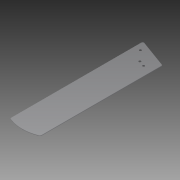
# Autodesk Inventor part: large ball holder
Saved by Autodesk Inventor 2014 SP1 (Build 180222100, 222)
## iProperties
Created: 2014-04-15
Part Number: large ball holder
Material: Generic
Document SubType Name: Modeling
Designer: Ryan
Density: 1 g/cm^3
Appearance: Polycarbonate - Clear
Author: Ryan
Autodesk Inventor part; units mm, degrees
ref_plane "YZ Plane" through (0, 0, 0) normal (1, 0, 0) x (0, 1, 0)
ref_plane "XZ Plane" through (0, 0, 0) normal (0, 1, 0) x (-1, 0, 0)
ref_plane "XY Plane" through (0, 0, 0) normal (0, 0, 1) x (1, 0, 0)
sketch "Sketch1" plane through (0, 0, 0) normal (0, 1, 0) x (-1, 0, 0)
  line L0 (27.8561, -123.3839) -> (27.8561, 130.6161)
  line L1 (27.8561, 130.6161) -> (-35.6439, 130.6161) construction
  line L2 (-35.6439, 130.6161) -> (-35.6439, -123.3839)
  line L3 (27.8561, -146.496) -> (-35.6439, -123.3839)
  line L4 (27.8561, -146.496) -> (27.8561, -123.3839)
  arc A0 (27.8561, 130.6161) -> (-35.6439, 130.6161) centre (-3.8939, 58.7362) ccw
  line L5 (-35.6439, -123.3839) -> (-3.8939, -52.0908)
  point P0 (0, 0)
  dimension "d3" = 254
  dimension "d4" = 110
  dimension "d6" = 78.5798
  dimension "d24" = 24.006
  constraints: 12 end point, 2 parallel, 2 point on circle, 1 centre point
  measures "d3" distance of L1.end L2.end
  measures "d4" angle of L3 L2
  measures "d6" radius of A0
  measures "d24" angle of L2 L5
extrude "Extrusion1" add sketch "Sketch1" along normal blind 1.5875
fillet "Fillet1" radius 3.175 4 edges at (-27.8561, 0.7937, -146.496) (35.6439, 0.7937, -123.3839) (35.6439, 0.7937, 130.6161) (-27.8561, 0.7937, 130.6161)
fillet "Fillet2" radius 0.635 16 edges at (-27.3175, 1.5875, 130.2862) (3.8939, 1.5875, 137.316) (35.1052, 1.5875, 130.2862) (35.6439, 1.5875, 3.6781) (35.0697, 1.5875, -122.9818) (4.9798, 1.5875, -134.5447) (-26.5022, 1.5875, -144.5624) (-27.8561, 1.5875, 2.5665) (-26.5022, 0, -144.5624) (4.9798, 0, -134.5447) (35.0697, 0, -122.9818) (35.6439, 0, 3.6781) (35.1052, 0, 130.2862) (3.8939, 0, 137.316) (-27.3175, 0, 130.2862) (-27.8561, 0, 2.5665)
sketch "Sketch3" plane through (0, 0, 0) normal (0, -1, 0) x (1, 0, 0)
  circle A0 centre (10.8789, -105.1316) radius 2.3114 projected
  circle A1 centre (-14.5211, -117.8316) radius 2.3114 projected
  circle A2 centre (23.5789, -105.1316) radius 2.3114 projected
  arc A3 (-27.2211, -141.9616) -> (-23.8124, -144.3485) centre (-24.6811, -141.9616) ccw projected
  line L0 (33.3376, -123.5476) -> (-23.8124, -144.3485) projected
  arc A4 (33.3376, -123.5476) -> (35.0089, -121.1607) centre (32.4689, -121.1607) ccw projected
  line L1 (35.0089, 128.5169) -> (35.0089, -121.1607) projected
  arc A5 (35.0089, 128.5169) -> (33.4314, 130.8675) centre (32.4689, 128.5169) ccw projected
  arc A6 (33.4314, 130.8675) -> (-25.6437, 130.8675) centre (3.8939, 58.7362) ccw projected
  arc A7 (-25.6437, 130.8675) -> (-27.2211, 128.5169) centre (-24.6811, 128.5169) ccw projected
  line L2 (-27.2211, -141.9616) -> (-27.2211, 128.5169) projected
  line L3 (32.4689, -121.1607) -> (15.1752, -73.6466)
  point P0 (0, 0)
  dimension "d39" = 20
  constraints: 2 end point
  measures "d39" angle of L1 L3
sketch "Sketch4" plane through (0, 0, 0) normal (0, -1, 0) x (0.9397, 0, 0.342)
  line L0 (-10.9286, -127.4989) -> (-71.7464, -127.4989) projected
  line L1 (-74.1332, -124.0901) -> (18.3759, 130.0766) projected
  circle A0 centre (-57.2364, -114.7989) radius 2.3114
  line L2 (-10.9286, -124.9589) -> (-10.9286, -74.3954) construction
  line L3 (-10.9286, -124.9589) -> (-35.7001, -124.9589) construction
  circle A1 centre (-57.2364, -102.0989) radius 2.3114
  circle A2 centre (-57.2364, -89.3989) radius 2.3114
  circle A3 centre (-44.5364, -114.7989) radius 2.3114
  circle A4 centre (-44.5364, -102.0989) radius 2.3114
  circle A5 centre (-44.5364, -89.3989) radius 2.3114
  circle A6 centre (-31.8364, -114.7989) radius 2.3114
  circle A7 centre (-31.8364, -102.0989) radius 2.3114
  circle A8 centre (-31.8364, -89.3989) radius 2.3114
  circle A9 centre (-19.1364, -114.7989) radius 2.3114
  circle A10 centre (-19.1364, -102.0989) radius 2.3114
  circle A11 centre (-19.1364, -89.3989) radius 2.3114
  circle A12 centre (-6.4364, -114.7989) radius 2.3114
  circle A13 centre (-6.4364, -102.0989) radius 2.3114
  circle A14 centre (-6.4364, -89.3989) radius 2.3114
  point P0 (0, 0)
  dimension "d26" = 4.6228
  dimension "d27" = 12.7
  dimension "d28" = 12.7
  dimension "d31" = 12.7
  dimension "d34" = 12.7
  constraints: 15 centre point, 2 end point, 1 horizontal, 1 perpendicular, 1 vertical, 28 other
  measures "d26" diameter of A0
  measures "d27" distance from line of L0 A0.centre
  measures "d28" distance from line of L1 A0.centre
  measures "d31" distance of A0.centre A1.centre
  measures "d34" distance of A0.centre A3.centre
extrude "Extrusion3" cut sketch "Sketch4" against normal blind 25.4 contours A0 | A7 | A10
body "Solid1"
